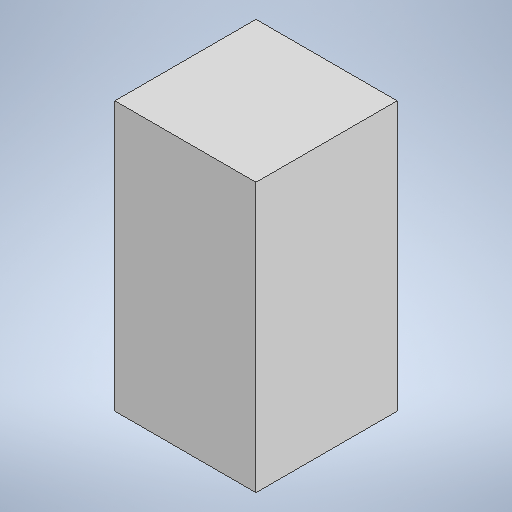
# Autodesk Inventor part: Air_heater_button
Saved by Autodesk Inventor 2025.2 (Build 292293000, 293)
## iProperties
Created: 2025-09-19
Part Number: Air_heater_button
Material: Generic
Document SubType Name: Modeling
Designer: TSO
Density: 1 g/cm^3
Appearance: Default
Author: TSO
Autodesk Inventor part; units mm, degrees
ref_plane "YZ Plane" through (0, 0, 0) normal (1, 0, 0) x (0, 1, 0)
ref_plane "XZ Plane" through (0, 0, 0) normal (0, 1, 0) x (-1, 0, 0)
ref_plane "XY Plane" through (0, 0, 0) normal (0, 0, 1) x (1, 0, 0)
sketch "Sketch1" plane through (0, 0, 0) normal (0, 1, 0) x (-1, 0, 0)
  line L0 (0, 0) -> (10.5, 0)
  line L1 (10.5, 0) -> (10.5, -10.5)
  line L2 (10.5, -10.5) -> (0, -10.5)
  line L3 (0, -10.5) -> (0, 0)
  dimension "d0" = 10.5
  dimension "d1" = 10.5
  constraints: 8 end point, 2 parallel, 1 horizontal, 1 perpendicular
  measures "d0" distance of L1.end L2.end
  measures "d1" distance of L0.end L1.end
extrude "Extrusion1" add sketch "Sketch1" along normal blind 20
body "Solid1"
